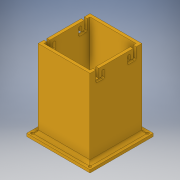
# Autodesk Inventor part: bateryHolder2.0
Saved by Autodesk Inventor 2017 (Build 210142000, 142)
## iProperties
Created: 2018-01-06
Part Number: bateryHolder2.0
Material: Generic
Document SubType Name: Modeling
Designer: User
Density: 1 g/cm^3
Appearance: Default(1)
Author: User
Autodesk Inventor part; units mm, degrees
ref_plane "YZ Plane" through (0, 0, 0) normal (1, 0, 0) x (0, 1, 0)
ref_plane "XZ Plane" through (0, 0, 0) normal (0, 1, 0) x (-1, 0, 0)
ref_plane "XY Plane" through (0, 0, 0) normal (0, 0, 1) x (1, 0, 0)
sketch "Sketch1" plane through (0, 0, 0) normal (0, 1, 0) x (-1, 0, 0)
  line L0 (0, 0) -> (50.8, 0)
  line L1 (50.8, 0) -> (50.8, -50.8)
  line L2 (50.8, -50.8) -> (0, -50.8)
  line L3 (0, -50.8) -> (0, 0)
  line L4 (53.975, 0) -> (53.975, 3.175)
  line L5 (53.975, 3.175) -> (50.8, 3.175)
  line L6 (-3.175, -50.8) -> (-3.175, -53.975)
  line L7 (-3.175, -53.975) -> (0, -53.975)
  line L8 (-3.175, -53.975) -> (53.975, -53.975)
  line L9 (53.975, -53.975) -> (53.975, 3.175)
  line L10 (53.975, 3.175) -> (-3.175, 3.175)
  line L11 (-3.175, 3.175) -> (-3.175, -53.975)
  line L12 (6.35, -6.35) -> (44.45, -6.35)
  line L13 (44.45, -6.35) -> (44.45, -44.45)
  line L14 (44.45, -44.45) -> (6.35, -44.45)
  line L15 (6.35, -44.45) -> (6.35, -6.35)
  line L16 (60.325, 9.525) -> (-9.525, 9.525)
  line L17 (-9.525, 9.525) -> (-9.525, -60.325)
  line L18 (-9.525, -60.325) -> (60.325, -60.325)
  line L19 (60.325, -60.325) -> (60.325, 9.525)
  dimension "d20" = 50.8
  dimension "d21" = 50.8
  dimension "d22" = 6.35
  dimension "d23" = 3.175
  dimension "d24" = 3.175
  dimension "d25" = 3.175
  dimension "d26" = 3.175
  dimension "d27" = 6.35
  dimension "d28" = 6.35
  dimension "d29" = 6.35
  dimension "d34" = 6.35
  dimension "d35" = 6.35
  dimension "d36" = 6.35
  dimension "d37" = 6.35
  constraints: 40 end point, 8 parallel, 4 horizontal, 4 perpendicular
  measures "d20" distance between parallel lines of L3 L1
  measures "d21" distance between parallel lines of L2 L0
  measures "d22" distance between parallel lines of L2 L14
  measures "d23" distance between parallel lines of L8 L2
  measures "d24" distance between parallel lines of L11 L3
  measures "d25" distance between parallel lines of L0 L10
  measures "d26" distance between parallel lines of L1 L9
  measures "d27" distance between parallel lines of L1 L13
  measures "d28" distance between parallel lines of L0 L12
  measures "d29" distance between parallel lines of L3 L15
  measures "d34" distance between parallel lines of L19 L9
  measures "d35" distance between parallel lines of L18 L8
  measures "d36" distance between parallel lines of L10 L16
  measures "d37" distance between parallel lines of L17 L11
extrude "Extrusion1" add sketch "Sketch1" along normal blind 88.9 contours L9 L8 L7 L6 L11 L10 L5 L4
sketch "Sketch2" plane through (3.175, 0, 3.175) normal (1, 0, 0) x (0, 0, -1)
  line L0 (3.175, 88.9) -> (53.975, 88.9) projected
  line L1 (50.8, 88.9) -> (47.625, 88.9)
  line L2 (47.625, 88.9) -> (47.625, 79.375)
  line L3 (49.0354, 76.2) -> (50.8, 76.2)
  line L4 (50.8, 76.2) -> (50.8, 88.9)
  line L5 (49.0354, 76.2) -> (41.275, 76.2)
  line L6 (41.275, 76.2) -> (41.275, 104.1556)
  line L7 (44.45, 79.375) -> (47.625, 79.375)
  line L8 (41.275, 76.2) -> (45.1552, 76.2)
  line L9 (44.45, 79.375) -> (44.45, 85.725)
  line L10 (44.45, 85.725) -> (41.275, 85.725)
  line L11 (41.275, 85.725) -> (41.275, 76.2)
  line L12 (57.15, 0) -> (57.15, 88.9) projected
  point P0 (3.175, 0)
  dimension "d10" = 3.175
  dimension "d11" = 6.35
  dimension "d12" = 9.525
  dimension "d13" = 3.175
  dimension "d14" = 3.175
  dimension "d15" = 3.175
  dimension "d16" = 12.7
  constraints: 22 end point, 5 parallel, 3 horizontal, 3 perpendicular, 1 point on line
  measures "d10" distance between parallel lines of L4 L2
  measures "d11" distance between parallel lines of L12 L4
  measures "d12" distance between parallel lines of L4 L11
  measures "d13" distance between parallel lines of L9 L11
  measures "d14" distance from line of L3.start L7
  measures "d15" distance between parallel lines of L0 L10
  measures "d16" distance between parallel lines of L0 L5
ref_plane "Work Plane1" through (-53.975, 0, -25.4) normal (0, 0, 1) x (1, 0, 0)
extrude "Extrusion3" cut sketch "Sketch2" against normal blind 3.175 contours L0 L4 L3 L5 L6 L10 L9 L7 L2
ref_plane "Work Plane2" through (-25.4, 0, -53.975) normal (-1, 0, 0) x (0, 0, 1)
fillet "Fillet1" radius 1.5875 4 edges at (1.5875, 76.2, -38.1) (1.5875, 85.725, -38.1) (1.5875, 76.2, -47.625) (1.5875, 85.725, -41.275)
mirror "Mirror1" about plane through (-25.4, 0, -53.975) normal (-1, 0, 0) of "Extrusion3", "Fillet1"
mirror "Mirror2" about plane through (-53.975, 0, -25.4) normal (0, 0, 1) of "Extrusion3", "Fillet1", "Mirror1"
extrude "Extrusion5" add sketch "Sketch1" along normal blind 3.175 contours L0 L1 L2 L3
extrude "Extrusion6" add sketch "Sketch1" along normal blind 3.175 contours L19 L18 L17 L16
sketch "Sketch3" plane through (0, 3.175, 0) normal (0, 1, 0) x (1, 0, 0)
  line L0 (-53.975, -3.175) -> (3.175, -3.175) projected
  line L1 (3.175, 53.975) -> (-53.975, 53.975) projected
  line L2 (3.175, -3.175) -> (3.175, 53.975) projected
  line L3 (-53.975, -3.175) -> (3.175, -3.175) projected
  line L4 (-53.975, 53.975) -> (-53.975, -3.175) projected
  line L5 (-60.325, -9.525) -> (9.525, -9.525) projected
  line L6 (9.525, -9.525) -> (9.525, 60.325) projected
  line L7 (9.525, 60.325) -> (-60.325, 60.325) projected
  line L8 (-60.325, 60.325) -> (-60.325, -9.525) projected
  point P0 (0, 0)
  point P1 (-57.15, -6.35)
  point P2 (-57.15, 57.15)
  point P3 (6.35, 57.15)
  point P4 (6.35, -6.35)
  dimension "d40" = 3.175
  dimension "d41" = 3.175
  dimension "d42" = 3.175
  dimension "d43" = 3.175
  dimension "d44" = 3.175
  dimension "d45" = 3.175
  dimension "d46" = 3.175
  dimension "d47" = 3.175
  measures "d40" distance from line of L0 point (-57.15, -6.35)
  measures "d41" distance from line of point (-57.15, -6.35) L8
  measures "d42" distance from line of L8 point (-57.15, 57.15)
  measures "d43" distance from line of L7 point (-57.15, 57.15)
  measures "d44" distance from line of L6 point (6.35, 57.15)
  measures "d45" distance from line of L7 point (6.35, 57.15)
  measures "d46" distance from line of L6 point (6.35, -6.35)
  measures "d47" distance from line of L5 point (6.35, -6.35)
hole "Hole1" at (6.35, 3.175, 6.35) at (6.35, 3.175, -57.15) at (-57.15, 3.175, -57.15) at (-57.15, 3.175, 6.35) direction (0, -1, 0) diameter 3.175 depth 25.4 tip angle 118
fillet "Fillet2" radius 3.175 8 edges at (-25.4, 3.175, 3.175) (-53.975, 3.175, -25.4) (3.175, 3.175, -25.4) (-25.4, 3.175, -53.975) (-25.4, 3.175, -50.8) (0, 3.175, -25.4) (-50.8, 3.175, -25.4) (-25.4, 3.175, 0)
ref_plane "Work Plane3" through (-53.975, 0, -25.4) normal (0, 0, 1) x (1, 0, 0)
equation "\"d41\" = d40"
equation "\"d42\" = d40"
equation "\"d43\" = d41"
equation "\"d44\" = d40"
equation "\"d45\" = d40"
equation "\"d46\" = d40"
equation "\"d47\" = d40"
body "Solid1"
